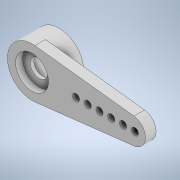
# Autodesk Inventor part: servo-horn-b
Saved by Autodesk Inventor 2020 (Build 240168000, 168)
## iProperties
Created: 2020-11-06
Part Number: servo-horn-b
Material: Generic
Document SubType Name: Modeling
Designer: alnwlsn
Density: 1 g/cm^3
Appearance: Default
Author: alnwlsn
Autodesk Inventor part; units mm, degrees
ref_plane "YZ Plane" through (0, 0, 0) normal (1, 0, 0) x (0, 1, 0)
ref_plane "XZ Plane" through (0, 0, 0) normal (0, 1, 0) x (-1, 0, 0)
ref_plane "XY Plane" through (0, 0, 0) normal (0, 0, 1) x (1, 0, 0)
sketch "Sketch1" plane through (0, 0, 0) normal (0, 0, 1) x (1, 0, 0)
  circle A0 centre (0, 0) radius 3.485
  arc A1 (14.4278, -1.8377) -> (14.4278, 1.8377) centre (14.215, 0) ccw
  line L0 (0.4008, 3.4619) -> (14.4278, 1.8377)
  line L1 (0.4008, -3.4619) -> (14.4278, -1.8377)
  line L2 (0, 0) -> (14.215, 0) construction
  line L3 (16.065, 5.1941) -> (16.065, -8.7582) construction
  line L4 (-3.485, 10.888) -> (-3.485, -12.1485) construction
  circle A2 centre (6.2317, 0) radius 0.5
  circle A3 centre (7.8983, 0) radius 0.5
  circle A4 centre (9.565, 0) radius 0.5
  circle A5 centre (11.2317, 0) radius 0.5
  circle A6 centre (12.8983, 0) radius 0.5
  circle A7 centre (14.565, 0) radius 0.5
  dimension "d1" = 19.55
  dimension "d2" = 1.85
  dimension "d3" = 6.97
  dimension "d4" = 1
  dimension "d7" = 1.6667
  dimension "d12" = 1.5
  constraints: 10 end point, 8 centre point, 6 tangent, 4 point on circle, 2 horizontal, 2 vertical, 1 coincident, 1 point on line, 10 other
  measures "d1" distance between parallel lines of L4 L3
  measures "d2" radius of A1
  measures "d3" diameter of A0
  measures "d4" diameter of A2
  measures "d7" distance of A2.centre A3.centre
  measures "d12" distance from line of L3 A7.centre
extrude "Extrusion1" add sketch "Sketch1" along normal blind 1.5
sketch "Sketch2" plane through (0, 0, 1.5) normal (0, 0, 1) x (1, 0, 0)
  arc A0 (0.4008, 3.4619) -> (0.4008, -3.4619) centre (0, 0) ccw projected
  circle A1 centre (0, 0) radius 1.25
  circle A2 centre (0, 0) radius 2.335
  dimension "d15" = 4.67
  dimension "d16" = 2.5
  constraints: 2 centre point, 2 coincident
  measures "d15" diameter of A2
  measures "d16" diameter of A1
extrude "Extrusion2" cut sketch "Sketch2" against normal blind 1.5 contours A1 | A2
sketch "Sketch3" plane through (0, 0, 0) normal (0, 0, -1) x (-1, 0, 0)
  circle A0 centre (0, 0) radius 2.335 projected
  circle A1 centre (0, 0) radius 3.485
  line L0 (-0.4008, -3.4619) -> (-14.4278, -1.8377) projected
  constraints: 1 coincident, 3 other
extrude "Extrusion3" add sketch "Sketch3" along normal blind 2.33
sketch "Sketch4" plane through (0, 0, 0) normal (0, 0, -1) x (-1, 0, 0)
  circle A0 centre (0, 0) radius 1.25
  circle A1 centre (0, 0) radius 3.485
  circle A2 centre (0, 0) radius 3.485 projected
  dimension "d21" = 2.5
  constraints: 2 centre point, 2 coincident, 1 concentric
  measures "d21" diameter of A0
extrude "Extrusion4" add sketch "Sketch4" against normal blind 0.5
body "Solid1"
